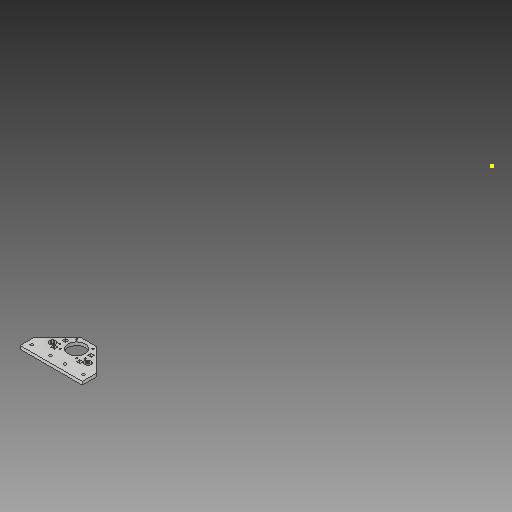
# Autodesk Inventor part: Rear Z Motor Mount
Saved by Autodesk Inventor 2018 (Build 220112000, 112)
## iProperties
Created: 2016-07-25
Part Number: Rear Z Motor Mount
Material: Generic
Document SubType Name: Modeling
Designer: User
Density: 1 g/cm^3
Appearance: Default
Author: User
Autodesk Inventor part; units mm, degrees
ref_plane "YZ Plane" through (0, 0, 0) normal (1, 0, 0) x (0, 1, 0)
ref_plane "XZ Plane" through (0, 0, 0) normal (0, 1, 0) x (-1, 0, 0)
ref_plane "XY Plane" through (0, 0, 0) normal (0, 0, 1) x (1, 0, 0)
sketch "Sketch1" plane through (0, 0, 0) normal (0, 1, 0) x (-1, 0, 0)
  line L0 (139.395291, 734.084292) -> (139.145335, 734.709338)
  line L1 (139.145335, 734.709338) -> (138.74531, 735.209285)
  line L2 (138.74531, 735.209285) -> (138.22032, 735.609261)
  line L3 (138.22032, 735.609261) -> (137.620314, 735.859289)
  line L4 (137.620314, 735.859289) -> (136.970314, 735.959304)
  line L5 (136.970314, 735.959304) -> (136.320293, 735.859285)
  line L6 (136.320293, 735.859285) -> (135.720329, 735.609258)
  line L7 (135.720329, 735.609258) -> (135.19531, 735.209292)
  line L8 (135.19531, 735.209292) -> (134.795318, 734.709302)
  line L9 (134.795318, 734.709302) -> (134.545299, 734.084298)
  line L10 (134.545299, 734.084298) -> (134.470282, 733.434297)
  line L11 (134.470282, 733.434297) -> (134.54536, 732.784303)
  line L12 (134.54536, 732.784303) -> (134.795378, 732.184363)
  line L13 (134.795378, 732.184363) -> (135.19537, 731.659309)
  line L14 (135.19537, 731.659309) -> (135.720373, 731.259323)
  line L15 (135.720373, 731.259323) -> (136.320343, 731.009311)
  line L16 (136.320343, 731.009311) -> (136.970367, 730.934291)
  line L17 (136.970367, 730.934291) -> (137.620418, 731.009376)
  line L18 (137.620418, 731.009376) -> (138.220418, 731.259419)
  line L19 (138.220418, 731.259419) -> (138.745325, 731.659299)
  line L20 (138.745325, 731.659299) -> (139.145329, 732.184326)
  line L21 (139.145329, 732.184326) -> (139.395338, 732.784288)
  line L22 (139.395338, 732.784288) -> (139.49533, 733.434137)
  line L23 (139.49533, 733.434137) -> (139.395291, 734.084292)
  line L24 (109.14464, 718.809311) -> (109.145998, 712.609302)
  line L25 (109.145998, 712.609302) -> (115.545973, 712.610704)
  line L26 (115.545973, 712.610704) -> (115.544615, 718.810713)
  line L27 (115.544615, 718.810713) -> (109.14464, 718.809311)
  line L28 (105.170214, 713.534161) -> (105.020247, 713.909169)
  line L29 (105.020247, 713.909169) -> (104.77027, 714.234177)
  line L30 (104.77027, 714.234177) -> (104.445291, 714.484219)
  line L31 (104.445291, 714.484219) -> (104.045334, 714.659273)
  line L32 (104.045334, 714.659273) -> (103.645324, 714.70929)
  line L33 (103.645324, 714.70929) -> (103.245335, 714.65927)
  line L34 (103.245335, 714.65927) -> (102.845343, 714.484247)
  line L35 (102.845343, 714.484247) -> (102.520335, 714.23427)
  line L36 (102.520335, 714.23427) -> (102.270303, 713.909305)
  line L37 (102.270303, 713.909305) -> (102.120296, 713.534313)
  line L38 (102.120296, 713.534313) -> (102.070277, 713.109272)
  line L39 (102.070277, 713.109272) -> (102.120296, 712.709294)
  line L40 (102.120296, 712.709294) -> (102.270268, 712.309311)
  line L41 (102.270268, 712.309311) -> (102.520266, 711.984276)
  line L42 (102.520266, 711.984276) -> (102.84521, 711.73426)
  line L43 (102.84521, 711.73426) -> (103.245165, 711.584114)
  line L44 (103.245165, 711.584114) -> (103.645165, 711.534098)
  line L45 (103.645165, 711.534098) -> (104.045186, 711.584122)
  line L46 (104.045186, 711.584122) -> (104.445183, 711.734099)
  line L47 (104.445183, 711.734099) -> (104.770183, 711.984071)
  line L48 (104.770183, 711.984071) -> (105.020236, 712.309063)
  line L49 (105.020236, 712.309063) -> (105.17037, 712.708985)
  line L50 (105.17037, 712.708985) -> (105.245245, 713.108394)
  line L51 (105.245245, 713.108394) -> (105.170214, 713.534161)
  line L52 (103.59529, 701.759382) -> (101.995303, 705.60938)
  line L53 (101.995303, 705.60938) -> (99.470328, 708.934371)
  line L54 (99.470328, 708.934371) -> (96.145337, 711.484388)
  line L55 (96.145337, 711.484388) -> (92.295319, 713.05936)
  line L56 (92.295319, 713.05936) -> (88.145309, 713.609327)
  line L57 (88.145309, 713.609327) -> (83.995304, 713.059318)
  line L58 (83.995304, 713.059318) -> (80.14528, 711.484306)
  line L59 (80.14528, 711.484306) -> (76.820289, 708.93429)
  line L60 (76.820289, 708.93429) -> (74.295314, 705.609299)
  line L61 (74.295314, 705.609299) -> (72.695283, 701.759319)
  line L62 (72.695283, 701.759319) -> (72.145316, 697.609313)
  line L63 (72.145316, 697.609313) -> (72.695283, 693.484285)
  line L64 (72.695283, 693.484285) -> (74.295314, 689.609285)
  line L65 (74.295314, 689.609285) -> (76.820289, 686.309314)
  line L66 (76.820289, 686.309314) -> (80.14528, 683.759298)
  line L67 (80.14528, 683.759298) -> (83.995282, 682.159257)
  line L68 (83.995282, 682.159257) -> (88.145293, 681.60929)
  line L69 (88.145293, 681.60929) -> (92.295298, 682.159299)
  line L70 (92.295298, 682.159299) -> (96.1453, 683.759288)
  line L71 (96.1453, 683.759288) -> (99.470291, 686.309304)
  line L72 (99.470291, 686.309304) -> (101.995266, 689.609275)
  line L73 (101.995266, 689.609275) -> (103.595297, 693.484276)
  line L74 (103.595297, 693.484276) -> (104.14532, 697.609224)
  line L75 (104.14532, 697.609224) -> (103.59529, 701.759382)
  line L76 (113.895233, 705.508847) -> (113.745267, 705.883856)
  line L77 (113.745267, 705.883856) -> (113.520146, 706.209334)
  line L78 (113.520146, 706.209334) -> (113.195174, 706.459372)
  line L79 (113.195174, 706.459372) -> (112.845114, 706.634306)
  line L80 (112.845114, 706.634306) -> (112.445132, 706.709288)
  line L81 (112.445132, 706.709288) -> (112.045113, 706.684282)
  line L82 (112.045113, 706.684282) -> (111.670099, 706.559312)
  line L83 (111.670099, 706.559312) -> (111.320076, 706.359366)
  line L84 (111.320076, 706.359366) -> (111.045103, 706.059375)
  line L85 (111.045103, 706.059375) -> (110.870168, 705.709315)
  line L86 (110.870168, 705.709315) -> (110.770262, 705.309317)
  line L87 (110.770262, 705.309317) -> (110.77035, 704.909299)
  line L88 (110.77035, 704.909299) -> (110.870426, 704.534322)
  line L89 (110.870426, 704.534322) -> (111.04538, 704.184315)
  line L90 (111.04538, 704.184315) -> (111.320343, 703.884272)
  line L91 (111.320343, 703.884272) -> (111.670328, 703.659241)
  line L92 (111.670328, 703.659241) -> (112.045299, 703.534186)
  line L93 (112.045299, 703.534186) -> (112.445314, 703.50911)
  line L94 (112.445314, 703.50911) -> (112.845294, 703.584062)
  line L95 (112.845294, 703.584062) -> (113.195352, 703.759042)
  line L96 (113.195352, 703.759042) -> (113.520346, 704.009009)
  line L97 (113.520346, 704.009009) -> (113.745232, 704.333827)
  line L98 (113.745232, 704.333827) -> (113.895239, 704.708819)
  line L99 (113.895239, 704.708819) -> (113.945257, 705.108829)
  line L100 (113.945257, 705.108829) -> (113.895233, 705.508847)
  line L101 (109.14464, 697.609313) -> (109.145998, 691.409304)
  line L102 (109.145998, 691.409304) -> (115.545973, 691.410706)
  line L103 (115.545973, 691.410706) -> (115.544615, 697.610715)
  line L104 (115.544615, 697.610715) -> (109.14464, 697.609313)
  line L105 (105.16778, 682.533999) -> (105.017813, 682.909007)
  line L106 (105.017813, 682.909007) -> (104.767857, 683.233987)
  line L107 (104.767857, 683.233987) -> (104.442857, 683.484046)
  line L108 (104.442857, 683.484046) -> (104.0429, 683.6591)
  line L109 (104.0429, 683.6591) -> (103.642836, 683.709124)
  line L110 (103.642836, 683.709124) -> (103.242842, 683.659103)
  line L111 (103.242842, 683.659103) -> (102.84285, 683.48408)
  line L112 (102.84285, 683.48408) -> (102.517822, 683.234087)
  line L113 (102.517822, 683.234087) -> (102.26781, 682.909149)
  line L114 (102.26781, 682.909149) -> (102.117803, 682.534157)
  line L115 (102.117803, 682.534157) -> (102.042746, 682.108654)
  line L116 (102.042746, 682.108654) -> (102.117675, 681.708798)
  line L117 (102.117675, 681.708798) -> (102.267647, 681.308815)
  line L118 (102.267647, 681.308815) -> (102.517645, 680.983781)
  line L119 (102.517645, 680.983781) -> (102.84261, 680.733749)
  line L120 (102.84261, 680.733749) -> (103.242551, 680.583608)
  line L121 (103.242551, 680.583608) -> (103.642546, 680.533593)
  line L122 (103.642546, 680.533593) -> (104.042561, 680.583616)
  line L123 (104.042561, 680.583616) -> (104.442544, 680.733588)
  line L124 (104.442544, 680.733588) -> (104.767565, 680.983576)
  line L125 (104.767565, 680.983576) -> (105.017618, 681.308568)
  line L126 (105.017618, 681.308568) -> (105.167752, 681.70849)
  line L127 (105.167752, 681.70849) -> (105.242752, 682.108567)
  line L128 (105.242752, 682.108567) -> (105.16778, 682.533999)
  line L129 (74.171005, 682.534425) -> (74.021036, 682.90944)
  line L130 (74.021036, 682.90944) -> (73.771079, 683.234421)
  line L131 (73.771079, 683.234421) -> (73.446094, 683.484469)
  line L132 (73.446094, 683.484469) -> (73.0461, 683.659538)
  line L133 (73.0461, 683.659538) -> (72.646127, 683.709551)
  line L134 (72.646127, 683.709551) -> (72.246112, 683.659528)
  line L135 (72.246112, 683.659528) -> (71.846138, 683.484513)
  line L136 (71.846138, 683.484513) -> (71.521096, 683.234509)
  line L137 (71.521096, 683.234509) -> (71.271076, 682.909561)
  line L138 (71.271076, 682.909561) -> (71.121072, 682.534576)
  line L139 (71.121072, 682.534576) -> (71.046082, 682.109455)
  line L140 (71.046082, 682.109455) -> (71.121043, 681.70943)
  line L141 (71.121043, 681.70943) -> (71.271013, 681.309455)
  line L142 (71.271013, 681.309455) -> (71.521019, 680.98441)
  line L143 (71.521019, 680.98441) -> (71.845997, 680.734367)
  line L144 (71.845997, 680.734367) -> (72.245919, 680.584234)
  line L145 (72.245919, 680.584234) -> (72.645863, 680.534224)
  line L146 (72.645863, 680.534224) -> (73.045836, 680.584243)
  line L147 (73.045836, 680.584243) -> (73.445857, 680.734229)
  line L148 (73.445857, 680.734229) -> (73.770864, 680.984206)
  line L149 (73.770864, 680.984206) -> (74.020917, 681.309198)
  line L150 (74.020917, 681.309198) -> (74.171053, 681.709127)
  line L151 (74.171053, 681.709127) -> (74.245995, 682.108893)
  line L152 (74.245995, 682.108893) -> (74.171005, 682.534425)
  line L153 (60.744623, 697.609313) -> (60.745981, 691.409304)
  line L154 (60.745981, 691.409304) -> (67.145601, 691.410706)
  line L155 (67.145601, 691.410706) -> (67.144243, 697.610715)
  line L156 (67.144243, 697.610715) -> (60.744623, 697.609313)
  line L157 (65.445222, 705.708927) -> (65.245261, 706.058976)
  line L158 (65.245261, 706.058976) -> (64.970319, 706.358996)
  line L159 (64.970319, 706.358996) -> (64.620368, 706.559031)
  line L160 (64.620368, 706.559031) -> (64.245365, 706.684097)
  line L161 (64.245365, 706.684097) -> (63.845371, 706.709172)
  line L162 (63.845371, 706.709172) -> (63.445342, 706.63421)
  line L163 (63.445342, 706.63421) -> (63.095318, 706.459248)
  line L164 (63.095318, 706.459248) -> (62.770303, 706.209264)
  line L165 (62.770303, 706.209264) -> (62.545319, 705.884305)
  line L166 (62.545319, 705.884305) -> (62.395309, 705.509305)
  line L167 (62.395309, 705.509305) -> (62.34529, 705.109286)
  line L168 (62.34529, 705.109286) -> (62.395309, 704.709311)
  line L169 (62.395309, 704.709311) -> (62.545278, 704.334295)
  line L170 (62.545278, 704.334295) -> (62.770227, 704.009267)
  line L171 (62.770227, 704.009267) -> (63.095178, 703.759245)
  line L172 (63.095178, 703.759245) -> (63.445158, 703.584151)
  line L173 (63.445158, 703.584151) -> (63.845174, 703.509162)
  line L174 (63.845174, 703.509162) -> (64.245172, 703.534167)
  line L175 (64.245172, 703.534167) -> (64.620197, 703.659124)
  line L176 (64.620197, 703.659124) -> (64.970184, 703.884119)
  line L177 (64.970184, 703.884119) -> (65.245179, 704.184133)
  line L178 (65.245179, 704.184133) -> (65.44522, 704.534094)
  line L179 (65.44522, 704.534094) -> (65.545248, 704.909083)
  line L180 (65.545248, 704.909083) -> (65.54516, 705.308937)
  line L181 (65.54516, 705.308937) -> (65.445222, 705.708927)
  line L182 (60.720321, 711.359386) -> (60.120286, 712.809328)
  line L183 (60.120286, 712.809328) -> (59.170321, 714.034334)
  line L184 (59.170321, 714.034334) -> (57.920292, 714.984294)
  line L185 (57.920292, 714.984294) -> (56.470304, 715.584314)
  line L186 (56.470304, 715.584314) -> (54.920313, 715.809279)
  line L187 (54.920313, 715.809279) -> (53.3703, 715.584314)
  line L188 (53.3703, 715.584314) -> (51.920324, 714.984265)
  line L189 (51.920324, 714.984265) -> (50.695291, 714.03428)
  line L190 (50.695291, 714.03428) -> (49.720286, 712.80929)
  line L191 (49.720286, 712.80929) -> (49.120279, 711.359335)
  line L192 (49.120279, 711.359335) -> (48.920291, 709.809301)
  line L193 (48.920291, 709.809301) -> (49.120279, 708.234289)
  line L194 (49.120279, 708.234289) -> (49.720286, 706.809312)
  line L195 (49.720286, 706.809312) -> (50.695291, 705.559302)
  line L196 (50.695291, 705.559302) -> (51.920324, 704.609274)
  line L197 (51.920324, 704.609274) -> (53.370281, 704.009266)
  line L198 (53.370281, 704.009266) -> (54.920295, 703.809281)
  line L199 (54.920295, 703.809281) -> (56.470286, 704.009271)
  line L200 (56.470286, 704.009271) -> (57.920231, 704.609308)
  line L201 (57.920231, 704.609308) -> (59.170193, 705.5594)
  line L202 (59.170193, 705.5594) -> (60.120153, 706.809429)
  line L203 (60.120153, 706.809429) -> (60.720131, 708.234419)
  line L204 (60.720131, 708.234419) -> (60.920304, 709.809457)
  line L205 (60.920304, 709.809457) -> (60.720321, 711.359386)
  line L206 (60.744623, 718.809311) -> (60.745981, 712.609302)
  line L207 (60.745981, 712.609302) -> (67.145956, 712.610704)
  line L208 (67.145956, 712.610704) -> (67.144598, 718.810713)
  line L209 (67.144598, 718.810713) -> (60.744623, 718.809311)
  line L210 (74.170237, 713.534159) -> (74.020268, 713.909175)
  line L211 (74.020268, 713.909175) -> (73.77029, 714.234182)
  line L212 (73.77029, 714.234182) -> (73.445325, 714.484214)
  line L213 (73.445325, 714.484214) -> (73.045332, 714.659284)
  line L214 (73.045332, 714.659284) -> (72.645364, 714.709296)
  line L215 (72.645364, 714.709296) -> (72.245354, 714.659273)
  line L216 (72.245354, 714.659273) -> (71.84538, 714.484258)
  line L217 (71.84538, 714.484258) -> (71.520359, 714.23427)
  line L218 (71.520359, 714.23427) -> (71.270319, 713.909295)
  line L219 (71.270319, 713.909295) -> (71.120314, 713.53431)
  line L220 (71.120314, 713.53431) -> (71.070296, 713.109272)
  line L221 (71.070296, 713.109272) -> (71.120314, 712.709296)
  line L222 (71.120314, 712.709296) -> (71.270284, 712.309321)
  line L223 (71.270284, 712.309321) -> (71.52029, 711.984276)
  line L224 (71.52029, 711.984276) -> (71.845248, 711.734249)
  line L225 (71.845248, 711.734249) -> (72.245184, 711.58411)
  line L226 (72.245184, 711.58411) -> (72.645205, 711.534091)
  line L227 (72.645205, 711.534091) -> (73.045183, 711.58411)
  line L228 (73.045183, 711.58411) -> (73.445218, 711.734102)
  line L229 (73.445218, 711.734102) -> (73.770204, 711.984063)
  line L230 (73.770204, 711.984063) -> (74.020258, 712.309055)
  line L231 (74.020258, 712.309055) -> (74.170394, 712.708984)
  line L232 (74.170394, 712.708984) -> (74.245268, 713.108391)
  line L233 (74.245268, 713.108391) -> (74.170237, 713.534159)
  line L234 (76.595279, 734.084304) -> (76.345325, 734.709343)
  line L235 (76.345325, 734.709343) -> (75.9453, 735.20929)
  line L236 (75.9453, 735.20929) -> (75.420297, 735.609276)
  line L237 (75.420297, 735.609276) -> (74.820291, 735.859304)
  line L238 (74.820291, 735.859304) -> (74.170311, 735.959315)
  line L239 (74.170311, 735.959315) -> (73.520311, 735.8593)
  line L240 (73.520311, 735.8593) -> (72.920297, 735.609251)
  line L241 (72.920297, 735.609251) -> (72.395278, 735.209286)
  line L242 (72.395278, 735.209286) -> (71.995303, 734.709317)
  line L243 (71.995303, 734.709317) -> (71.745278, 734.084298)
  line L244 (71.745278, 734.084298) -> (71.670261, 733.434297)
  line L245 (71.670261, 733.434297) -> (71.745339, 732.784303)
  line L246 (71.745339, 732.784303) -> (71.995364, 732.184347)
  line L247 (71.995364, 732.184347) -> (72.395339, 731.659315)
  line L248 (72.395339, 731.659315) -> (72.920342, 731.259329)
  line L249 (72.920342, 731.259329) -> (73.520349, 731.009301)
  line L250 (73.520349, 731.009301) -> (74.170352, 730.934284)
  line L251 (74.170352, 730.934284) -> (74.820324, 731.009359)
  line L252 (74.820324, 731.009359) -> (75.420324, 731.259402)
  line L253 (75.420324, 731.259402) -> (75.945286, 731.659324)
  line L254 (75.945286, 731.659324) -> (76.34529, 732.184351)
  line L255 (76.34529, 732.184351) -> (76.595297, 732.784306)
  line L256 (76.595297, 732.784306) -> (76.695302, 733.434247)
  line L257 (76.695302, 733.434247) -> (76.595279, 734.084304)
  line L258 (104.570192, 734.084233) -> (104.320241, 734.709264)
  line L259 (104.320241, 734.709264) -> (103.920208, 735.209222)
  line L260 (103.920208, 735.209222) -> (103.395205, 735.609208)
  line L261 (103.395205, 735.609208) -> (102.770266, 735.859201)
  line L262 (102.770266, 735.859201) -> (102.120287, 735.959212)
  line L263 (102.120287, 735.959212) -> (101.470244, 735.859191)
  line L264 (101.470244, 735.859191) -> (100.845246, 735.609253)
  line L265 (100.845246, 735.609253) -> (100.320228, 735.209288)
  line L266 (100.320228, 735.209288) -> (99.920235, 734.709298)
  line L267 (99.920235, 734.709298) -> (99.670213, 734.084286)
  line L268 (99.670213, 734.084286) -> (99.570198, 733.434286)
  line L269 (99.570198, 733.434286) -> (99.670213, 732.784286)
  line L270 (99.670213, 732.784286) -> (99.920235, 732.184338)
  line L271 (99.920235, 732.184338) -> (100.320226, 731.659284)
  line L272 (100.320226, 731.659284) -> (100.845229, 731.259298)
  line L273 (100.845229, 731.259298) -> (101.4702, 731.009293)
  line L274 (101.4702, 731.009293) -> (102.120246, 730.934271)
  line L275 (102.120246, 730.934271) -> (102.770221, 731.009347)
  line L276 (102.770221, 731.009347) -> (103.395237, 731.259292)
  line L277 (103.395237, 731.259292) -> (103.920134, 731.659163)
  line L278 (103.920134, 731.659163) -> (104.320146, 732.184201)
  line L279 (104.320146, 732.184201) -> (104.570149, 732.784148)
  line L280 (104.570149, 732.784148) -> (104.670192, 733.434331)
  line L281 (104.670192, 733.434331) -> (104.570192, 734.084233)
  line L282 (41.745244, 734.084338) -> (41.495293, 734.70937)
  line L283 (41.495293, 734.70937) -> (41.095291, 735.209288)
  line L284 (41.095291, 735.209288) -> (40.570288, 735.609274)
  line L285 (40.570288, 735.609274) -> (39.970281, 735.859302)
  line L286 (39.970281, 735.859302) -> (39.320302, 735.959314)
  line L287 (39.320302, 735.959314) -> (38.670302, 735.859299)
  line L288 (38.670302, 735.859299) -> (38.070302, 735.609256)
  line L289 (38.070302, 735.609256) -> (37.545297, 735.209301)
  line L290 (37.545297, 735.209301) -> (37.145321, 734.709331)
  line L291 (37.145321, 734.709331) -> (36.895293, 734.084305)
  line L292 (36.895293, 734.084305) -> (36.795278, 733.434302)
  line L293 (36.795278, 733.434302) -> (36.895293, 732.784298)
  line L294 (36.895293, 732.784298) -> (37.145321, 732.184335)
  line L295 (37.145321, 732.184335) -> (37.545297, 731.659302)
  line L296 (37.545297, 731.659302) -> (38.070286, 731.259327)
  line L297 (38.070286, 731.259327) -> (38.670292, 731.009299)
  line L298 (38.670292, 731.009299) -> (39.320296, 730.934282)
  line L299 (39.320296, 730.934282) -> (39.970271, 731.009358)
  line L300 (39.970271, 731.009358) -> (40.570271, 731.259401)
  line L301 (40.570271, 731.259401) -> (41.09529, 731.659366)
  line L302 (41.09529, 731.659366) -> (41.495302, 732.184403)
  line L303 (41.495302, 732.184403) -> (41.745305, 732.78435)
  line L304 (41.745305, 732.78435) -> (41.820321, 733.434347)
  line L305 (41.820321, 733.434347) -> (41.745244, 734.084338)
  line L306 (29.317325, 745.634246) -> (29.323282, 718.434313)
  line L307 (29.323282, 718.434313) -> (72.657773, 675.118798)
  line L308 (72.657773, 675.118798) -> (103.657753, 675.125587)
  line L309 (103.657753, 675.125587) -> (146.973268, 718.460078)
  line L310 (146.973268, 718.460078) -> (146.967311, 745.66001)
  line L311 (146.967311, 745.66001) -> (29.317325, 745.634246)
  line L312 (127.170308, 711.359328) -> (126.570264, 712.809292)
  line L313 (126.570264, 712.809292) -> (125.595227, 714.03429)
  line L314 (125.595227, 714.03429) -> (124.370208, 714.984308)
  line L315 (124.370208, 714.984308) -> (122.920216, 715.584329)
  line L316 (122.920216, 715.584329) -> (121.370225, 715.809294)
  line L317 (121.370225, 715.809294) -> (119.820212, 715.584329)
  line L318 (119.820212, 715.584329) -> (118.370251, 714.984286)
  line L319 (118.370251, 714.984286) -> (117.120289, 714.034195)
  line L320 (117.120289, 714.034195) -> (116.170282, 712.809189)
  line L321 (116.170282, 712.809189) -> (115.570267, 711.359212)
  line L322 (115.570267, 711.359212) -> (115.370283, 709.809215)
  line L323 (115.370283, 709.809215) -> (115.570272, 708.234198)
  line L324 (115.570272, 708.234198) -> (116.170287, 706.809199)
  line L325 (116.170287, 706.809199) -> (117.120379, 705.559237)
  line L326 (117.120379, 705.559237) -> (118.370408, 704.609277)
  line L327 (118.370408, 704.609277) -> (119.820381, 704.009263)
  line L328 (119.820381, 704.009263) -> (121.370394, 703.809278)
  line L329 (121.370394, 703.809278) -> (122.920385, 704.009269)
  line L330 (122.920385, 704.009269) -> (124.370365, 704.60932)
  line L331 (124.370365, 704.60932) -> (125.595384, 705.559294)
  line L332 (125.595384, 705.559294) -> (126.570146, 706.809314)
  line L333 (126.570146, 706.809314) -> (127.170133, 708.234325)
  line L334 (127.170133, 708.234325) -> (127.370301, 709.809322)
  line L335 (127.370301, 709.809322) -> (127.170308, 711.359328)
  point P0 (0, 0)
  constraints: 672 end point, 122 parallel, 97 perpendicular
extrude "Extrusion1" add sketch "Sketch1" along normal blind 6 contours L281 L280 L279 L278 L277 L276 L275 L274 L273 L272 L271 L270 L269 L268 L267 L266 L265 L264 L263 L262 L261 L260 L259 L258 | L311 L310 L309 L308 L307 L306
sketch "Sketch2" plane through (0, 0, 0) normal (0, -1, 0) x (1, 0, 0)
  line L0 (-104.14532, 697.609224) -> (-103.59529, 701.759382)
  line L1 (-103.59529, 701.759382) -> (-101.995303, 705.60938)
  line L2 (-101.995303, 705.60938) -> (-99.470328, 708.934371)
  line L3 (-99.470328, 708.934371) -> (-96.145337, 711.484388)
  line L4 (-96.145337, 711.484388) -> (-92.295319, 713.05936)
  line L5 (-92.295319, 713.05936) -> (-88.145309, 713.609327)
  line L6 (-88.145309, 713.609327) -> (-83.995304, 713.059318)
  line L7 (-83.995304, 713.059318) -> (-80.14528, 711.484306)
  line L8 (-80.14528, 711.484306) -> (-76.820289, 708.93429)
  line L9 (-76.820289, 708.93429) -> (-74.295314, 705.609299)
  line L10 (-74.295314, 705.609299) -> (-72.695283, 701.759319)
  line L11 (-72.695283, 701.759319) -> (-72.145316, 697.609313)
  line L12 (-72.145316, 697.609313) -> (-72.695283, 693.484285)
  line L13 (-72.695283, 693.484285) -> (-74.295314, 689.609285)
  line L14 (-74.295314, 689.609285) -> (-76.820289, 686.309314)
  line L15 (-76.820289, 686.309314) -> (-80.14528, 683.759298)
  line L16 (-80.14528, 683.759298) -> (-83.995282, 682.159257)
  line L17 (-83.995282, 682.159257) -> (-88.145293, 681.60929)
  line L18 (-88.145293, 681.60929) -> (-92.295298, 682.159299)
  line L19 (-92.295298, 682.159299) -> (-96.1453, 683.759288)
  line L20 (-96.1453, 683.759288) -> (-99.470291, 686.309304)
  line L21 (-99.470291, 686.309304) -> (-101.995266, 689.609275)
  line L22 (-101.995266, 689.609275) -> (-103.595297, 693.484276)
  line L23 (-103.595297, 693.484276) -> (-104.14532, 697.609224)
  line L24 (-127.370301, 709.809322) -> (-127.170308, 711.359328)
  line L25 (-127.170308, 711.359328) -> (-126.570264, 712.809292)
  line L26 (-126.570264, 712.809292) -> (-125.595227, 714.03429)
  line L27 (-125.595227, 714.03429) -> (-124.370208, 714.984308)
  line L28 (-124.370208, 714.984308) -> (-122.920216, 715.584329)
  line L29 (-122.920216, 715.584329) -> (-121.370225, 715.809294)
  line L30 (-121.370225, 715.809294) -> (-119.820212, 715.584329)
  line L31 (-119.820212, 715.584329) -> (-118.370251, 714.984286)
  line L32 (-118.370251, 714.984286) -> (-117.120289, 714.034195)
  line L33 (-117.120289, 714.034195) -> (-116.170282, 712.809189)
  line L34 (-116.170282, 712.809189) -> (-115.570267, 711.359212)
  line L35 (-115.570267, 711.359212) -> (-115.370283, 709.809215)
  line L36 (-115.370283, 709.809215) -> (-115.570272, 708.234198)
  line L37 (-115.570272, 708.234198) -> (-116.170287, 706.809199)
  line L38 (-116.170287, 706.809199) -> (-117.120379, 705.559237)
  line L39 (-117.120379, 705.559237) -> (-118.370408, 704.609277)
  line L40 (-118.370408, 704.609277) -> (-119.820381, 704.009263)
  line L41 (-119.820381, 704.009263) -> (-121.370394, 703.809278)
  line L42 (-121.370394, 703.809278) -> (-122.920385, 704.009269)
  line L43 (-122.920385, 704.009269) -> (-124.370365, 704.60932)
  line L44 (-124.370365, 704.60932) -> (-125.595384, 705.559294)
  line L45 (-125.595384, 705.559294) -> (-126.570146, 706.809314)
  line L46 (-126.570146, 706.809314) -> (-127.170133, 708.234325)
  line L47 (-127.170133, 708.234325) -> (-127.370301, 709.809322)
  line L48 (-60.920304, 709.809457) -> (-60.720321, 711.359386)
  line L49 (-60.720321, 711.359386) -> (-60.120286, 712.809328)
  line L50 (-60.120286, 712.809328) -> (-59.170321, 714.034334)
  line L51 (-59.170321, 714.034334) -> (-57.920292, 714.984294)
  line L52 (-57.920292, 714.984294) -> (-56.470304, 715.584314)
  line L53 (-56.470304, 715.584314) -> (-54.920313, 715.809279)
  line L54 (-54.920313, 715.809279) -> (-53.3703, 715.584314)
  line L55 (-53.3703, 715.584314) -> (-51.920324, 714.984265)
  line L56 (-51.920324, 714.984265) -> (-50.695291, 714.03428)
  line L57 (-50.695291, 714.03428) -> (-49.720286, 712.80929)
  line L58 (-49.720286, 712.80929) -> (-49.120279, 711.359335)
  line L59 (-49.120279, 711.359335) -> (-48.920291, 709.809301)
  line L60 (-48.920291, 709.809301) -> (-49.120279, 708.234289)
  line L61 (-49.120279, 708.234289) -> (-49.720286, 706.809312)
  line L62 (-49.720286, 706.809312) -> (-50.695291, 705.559302)
  line L63 (-50.695291, 705.559302) -> (-51.920324, 704.609274)
  line L64 (-51.920324, 704.609274) -> (-53.370281, 704.009266)
  line L65 (-53.370281, 704.009266) -> (-54.920295, 703.809281)
  line L66 (-54.920295, 703.809281) -> (-56.470286, 704.009271)
  line L67 (-56.470286, 704.009271) -> (-57.920231, 704.609308)
  line L68 (-57.920231, 704.609308) -> (-59.170193, 705.5594)
  line L69 (-59.170193, 705.5594) -> (-60.120153, 706.809429)
  line L70 (-60.120153, 706.809429) -> (-60.720131, 708.234419)
  line L71 (-60.720131, 708.234419) -> (-60.920304, 709.809457)
  line L72 (-67.144598, 718.810713) -> (-60.744623, 718.809311)
  line L73 (-60.744623, 718.809311) -> (-60.745981, 712.609302)
  line L74 (-60.745981, 712.609302) -> (-67.145956, 712.610704)
  line L75 (-67.145956, 712.610704) -> (-67.144598, 718.810713)
  line L76 (-115.544615, 697.610715) -> (-109.14464, 697.609313)
  line L77 (-109.14464, 697.609313) -> (-109.145998, 691.409304)
  line L78 (-109.145998, 691.409304) -> (-115.545973, 691.410706)
  line L79 (-115.545973, 691.410706) -> (-115.544615, 697.610715)
  line L80 (-115.544615, 718.810713) -> (-109.14464, 718.809311)
  line L81 (-109.14464, 718.809311) -> (-109.145998, 712.609302)
  line L82 (-109.145998, 712.609302) -> (-115.545973, 712.610704)
  line L83 (-115.545973, 712.610704) -> (-115.544615, 718.810713)
  line L84 (-67.144243, 697.610715) -> (-60.744623, 697.609313)
  line L85 (-60.744623, 697.609313) -> (-60.745981, 691.409304)
  line L86 (-60.745981, 691.409304) -> (-67.145601, 691.410706)
  line L87 (-67.145601, 691.410706) -> (-67.144243, 697.610715)
  line L88 (-139.49533, 733.434137) -> (-139.395291, 734.084292)
  line L89 (-139.395291, 734.084292) -> (-139.145335, 734.709338)
  line L90 (-139.145335, 734.709338) -> (-138.74531, 735.209285)
  line L91 (-138.74531, 735.209285) -> (-138.22032, 735.609261)
  line L92 (-138.22032, 735.609261) -> (-137.620314, 735.859289)
  line L93 (-137.620314, 735.859289) -> (-136.970314, 735.959304)
  line L94 (-136.970314, 735.959304) -> (-136.320293, 735.859285)
  line L95 (-136.320293, 735.859285) -> (-135.720329, 735.609258)
  line L96 (-135.720329, 735.609258) -> (-135.19531, 735.209292)
  line L97 (-135.19531, 735.209292) -> (-134.795318, 734.709302)
  line L98 (-134.795318, 734.709302) -> (-134.545299, 734.084298)
  line L99 (-134.545299, 734.084298) -> (-134.470282, 733.434297)
  line L100 (-134.470282, 733.434297) -> (-134.54536, 732.784303)
  line L101 (-134.54536, 732.784303) -> (-134.795378, 732.184363)
  line L102 (-134.795378, 732.184363) -> (-135.19537, 731.659309)
  line L103 (-135.19537, 731.659309) -> (-135.720373, 731.259323)
  line L104 (-135.720373, 731.259323) -> (-136.320343, 731.009311)
  line L105 (-136.320343, 731.009311) -> (-136.970367, 730.934291)
  line L106 (-136.970367, 730.934291) -> (-137.620418, 731.009376)
  line L107 (-137.620418, 731.009376) -> (-138.220418, 731.259419)
  line L108 (-138.220418, 731.259419) -> (-138.745325, 731.659299)
  line L109 (-138.745325, 731.659299) -> (-139.145329, 732.184326)
  line L110 (-139.145329, 732.184326) -> (-139.395338, 732.784288)
  line L111 (-139.395338, 732.784288) -> (-139.49533, 733.434137)
  line L112 (-41.820321, 733.434347) -> (-41.745244, 734.084338)
  line L113 (-41.745244, 734.084338) -> (-41.495293, 734.70937)
  line L114 (-41.495293, 734.70937) -> (-41.095291, 735.209288)
  line L115 (-41.095291, 735.209288) -> (-40.570288, 735.609274)
  line L116 (-40.570288, 735.609274) -> (-39.970281, 735.859302)
  line L117 (-39.970281, 735.859302) -> (-39.320302, 735.959314)
  line L118 (-39.320302, 735.959314) -> (-38.670302, 735.859299)
  line L119 (-38.670302, 735.859299) -> (-38.070302, 735.609256)
  line L120 (-38.070302, 735.609256) -> (-37.545297, 735.209301)
  line L121 (-37.545297, 735.209301) -> (-37.145321, 734.709331)
  line L122 (-37.145321, 734.709331) -> (-36.895293, 734.084305)
  line L123 (-36.895293, 734.084305) -> (-36.795278, 733.434302)
  line L124 (-36.795278, 733.434302) -> (-36.895293, 732.784298)
  line L125 (-36.895293, 732.784298) -> (-37.145321, 732.184335)
  line L126 (-37.145321, 732.184335) -> (-37.545297, 731.659302)
  line L127 (-37.545297, 731.659302) -> (-38.070286, 731.259327)
  line L128 (-38.070286, 731.259327) -> (-38.670292, 731.009299)
  line L129 (-38.670292, 731.009299) -> (-39.320296, 730.934282)
  line L130 (-39.320296, 730.934282) -> (-39.970271, 731.009358)
  line L131 (-39.970271, 731.009358) -> (-40.570271, 731.259401)
  line L132 (-40.570271, 731.259401) -> (-41.09529, 731.659366)
  line L133 (-41.09529, 731.659366) -> (-41.495302, 732.184403)
  line L134 (-41.495302, 732.184403) -> (-41.745305, 732.78435)
  line L135 (-41.745305, 732.78435) -> (-41.820321, 733.434347)
  line L136 (-76.695302, 733.434247) -> (-76.595279, 734.084304)
  line L137 (-76.595279, 734.084304) -> (-76.345325, 734.709343)
  line L138 (-76.345325, 734.709343) -> (-75.9453, 735.20929)
  line L139 (-75.9453, 735.20929) -> (-75.420297, 735.609276)
  line L140 (-75.420297, 735.609276) -> (-74.820291, 735.859304)
  line L141 (-74.820291, 735.859304) -> (-74.170311, 735.959315)
  line L142 (-74.170311, 735.959315) -> (-73.520311, 735.8593)
  line L143 (-73.520311, 735.8593) -> (-72.920297, 735.609251)
  line L144 (-72.920297, 735.609251) -> (-72.395278, 735.209286)
  line L145 (-72.395278, 735.209286) -> (-71.995303, 734.709317)
  line L146 (-71.995303, 734.709317) -> (-71.745278, 734.084298)
  line L147 (-71.745278, 734.084298) -> (-71.670261, 733.434297)
  line L148 (-71.670261, 733.434297) -> (-71.745339, 732.784303)
  line L149 (-71.745339, 732.784303) -> (-71.995364, 732.184347)
  line L150 (-71.995364, 732.184347) -> (-72.395339, 731.659315)
  line L151 (-72.395339, 731.659315) -> (-72.920342, 731.259329)
  line L152 (-72.920342, 731.259329) -> (-73.520349, 731.009301)
  line L153 (-73.520349, 731.009301) -> (-74.170352, 730.934284)
  line L154 (-74.170352, 730.934284) -> (-74.820324, 731.009359)
  line L155 (-74.820324, 731.009359) -> (-75.420324, 731.259402)
  line L156 (-75.420324, 731.259402) -> (-75.945286, 731.659324)
  line L157 (-75.945286, 731.659324) -> (-76.34529, 732.184351)
  line L158 (-76.34529, 732.184351) -> (-76.595297, 732.784306)
  line L159 (-76.595297, 732.784306) -> (-76.695302, 733.434247)
  line L160 (-65.54516, 705.308937) -> (-65.445222, 705.708927)
  line L161 (-65.445222, 705.708927) -> (-65.245261, 706.058976)
  line L162 (-65.245261, 706.058976) -> (-64.970319, 706.358996)
  line L163 (-64.970319, 706.358996) -> (-64.620368, 706.559031)
  line L164 (-64.620368, 706.559031) -> (-64.245365, 706.684097)
  line L165 (-64.245365, 706.684097) -> (-63.845371, 706.709172)
  line L166 (-63.845371, 706.709172) -> (-63.445342, 706.63421)
  line L167 (-63.445342, 706.63421) -> (-63.095318, 706.459248)
  line L168 (-63.095318, 706.459248) -> (-62.770303, 706.209264)
  line L169 (-62.770303, 706.209264) -> (-62.545319, 705.884305)
  line L170 (-62.545319, 705.884305) -> (-62.395309, 705.509305)
  line L171 (-62.395309, 705.509305) -> (-62.34529, 705.109286)
  line L172 (-62.34529, 705.109286) -> (-62.395309, 704.709311)
  line L173 (-62.395309, 704.709311) -> (-62.545278, 704.334295)
  line L174 (-62.545278, 704.334295) -> (-62.770227, 704.009267)
  line L175 (-62.770227, 704.009267) -> (-63.095178, 703.759245)
  line L176 (-63.095178, 703.759245) -> (-63.445158, 703.584151)
  line L177 (-63.445158, 703.584151) -> (-63.845174, 703.509162)
  line L178 (-63.845174, 703.509162) -> (-64.245172, 703.534167)
  line L179 (-64.245172, 703.534167) -> (-64.620197, 703.659124)
  line L180 (-64.620197, 703.659124) -> (-64.970184, 703.884119)
  line L181 (-64.970184, 703.884119) -> (-65.245179, 704.184133)
  line L182 (-65.245179, 704.184133) -> (-65.44522, 704.534094)
  line L183 (-65.44522, 704.534094) -> (-65.545248, 704.909083)
  line L184 (-65.545248, 704.909083) -> (-65.54516, 705.308937)
  line L185 (-113.945257, 705.108829) -> (-113.895233, 705.508847)
  line L186 (-113.895233, 705.508847) -> (-113.745267, 705.883856)
  line L187 (-113.745267, 705.883856) -> (-113.520146, 706.209334)
  line L188 (-113.520146, 706.209334) -> (-113.195174, 706.459372)
  line L189 (-113.195174, 706.459372) -> (-112.845114, 706.634306)
  line L190 (-112.845114, 706.634306) -> (-112.445132, 706.709288)
  line L191 (-112.445132, 706.709288) -> (-112.045113, 706.684282)
  line L192 (-112.045113, 706.684282) -> (-111.670099, 706.559312)
  line L193 (-111.670099, 706.559312) -> (-111.320076, 706.359366)
  line L194 (-111.320076, 706.359366) -> (-111.045103, 706.059375)
  line L195 (-111.045103, 706.059375) -> (-110.870168, 705.709315)
  line L196 (-110.870168, 705.709315) -> (-110.770262, 705.309317)
  line L197 (-110.770262, 705.309317) -> (-110.77035, 704.909299)
  line L198 (-110.77035, 704.909299) -> (-110.870426, 704.534322)
  line L199 (-110.870426, 704.534322) -> (-111.04538, 704.184315)
  line L200 (-111.04538, 704.184315) -> (-111.320343, 703.884272)
  line L201 (-111.320343, 703.884272) -> (-111.670328, 703.659241)
  line L202 (-111.670328, 703.659241) -> (-112.045299, 703.534186)
  line L203 (-112.045299, 703.534186) -> (-112.445314, 703.50911)
  line L204 (-112.445314, 703.50911) -> (-112.845294, 703.584062)
  line L205 (-112.845294, 703.584062) -> (-113.195352, 703.759042)
  line L206 (-113.195352, 703.759042) -> (-113.520346, 704.009009)
  line L207 (-113.520346, 704.009009) -> (-113.745232, 704.333827)
  line L208 (-113.745232, 704.333827) -> (-113.895239, 704.708819)
  line L209 (-113.895239, 704.708819) -> (-113.945257, 705.108829)
  line L210 (-105.242752, 682.108567) -> (-105.16778, 682.533999)
  line L211 (-105.16778, 682.533999) -> (-105.017813, 682.909007)
  line L212 (-105.017813, 682.909007) -> (-104.767857, 683.233987)
  line L213 (-104.767857, 683.233987) -> (-104.442857, 683.484046)
  line L214 (-104.442857, 683.484046) -> (-104.0429, 683.6591)
  line L215 (-104.0429, 683.6591) -> (-103.642836, 683.709124)
  line L216 (-103.642836, 683.709124) -> (-103.242842, 683.659103)
  line L217 (-103.242842, 683.659103) -> (-102.84285, 683.48408)
  line L218 (-102.84285, 683.48408) -> (-102.517822, 683.234087)
  line L219 (-102.517822, 683.234087) -> (-102.26781, 682.909149)
  line L220 (-102.26781, 682.909149) -> (-102.117803, 682.534157)
  line L221 (-102.117803, 682.534157) -> (-102.042746, 682.108654)
  line L222 (-102.042746, 682.108654) -> (-102.117675, 681.708798)
  line L223 (-102.117675, 681.708798) -> (-102.267647, 681.308815)
  line L224 (-102.267647, 681.308815) -> (-102.517645, 680.983781)
  line L225 (-102.517645, 680.983781) -> (-102.84261, 680.733749)
  line L226 (-102.84261, 680.733749) -> (-103.242551, 680.583608)
  line L227 (-103.242551, 680.583608) -> (-103.642546, 680.533593)
  line L228 (-103.642546, 680.533593) -> (-104.042561, 680.583616)
  line L229 (-104.042561, 680.583616) -> (-104.442544, 680.733588)
  line L230 (-104.442544, 680.733588) -> (-104.767565, 680.983576)
  line L231 (-104.767565, 680.983576) -> (-105.017618, 681.308568)
  line L232 (-105.017618, 681.308568) -> (-105.167752, 681.70849)
  line L233 (-105.167752, 681.70849) -> (-105.242752, 682.108567)
  line L234 (-74.245995, 682.108893) -> (-74.171005, 682.534425)
  line L235 (-74.171005, 682.534425) -> (-74.021036, 682.90944)
  line L236 (-74.021036, 682.90944) -> (-73.771079, 683.234421)
  line L237 (-73.771079, 683.234421) -> (-73.446094, 683.484469)
  line L238 (-73.446094, 683.484469) -> (-73.0461, 683.659538)
  line L239 (-73.0461, 683.659538) -> (-72.646127, 683.709551)
  line L240 (-72.646127, 683.709551) -> (-72.246112, 683.659528)
  line L241 (-72.246112, 683.659528) -> (-71.846138, 683.484513)
  line L242 (-71.846138, 683.484513) -> (-71.521096, 683.234509)
  line L243 (-71.521096, 683.234509) -> (-71.271076, 682.909561)
  line L244 (-71.271076, 682.909561) -> (-71.121072, 682.534576)
  line L245 (-71.121072, 682.534576) -> (-71.046082, 682.109455)
  line L246 (-71.046082, 682.109455) -> (-71.121043, 681.70943)
  line L247 (-71.121043, 681.70943) -> (-71.271013, 681.309455)
  line L248 (-71.271013, 681.309455) -> (-71.521019, 680.98441)
  line L249 (-71.521019, 680.98441) -> (-71.845997, 680.734367)
  line L250 (-71.845997, 680.734367) -> (-72.245919, 680.584234)
  line L251 (-72.245919, 680.584234) -> (-72.645863, 680.534224)
  line L252 (-72.645863, 680.534224) -> (-73.045836, 680.584243)
  line L253 (-73.045836, 680.584243) -> (-73.445857, 680.734229)
  line L254 (-73.445857, 680.734229) -> (-73.770864, 680.984206)
  line L255 (-73.770864, 680.984206) -> (-74.020917, 681.309198)
  line L256 (-74.020917, 681.309198) -> (-74.171053, 681.709127)
  line L257 (-74.171053, 681.709127) -> (-74.245995, 682.108893)
  line L258 (-74.245268, 713.108391) -> (-74.170237, 713.534159)
  line L259 (-74.170237, 713.534159) -> (-74.020268, 713.909175)
  line L260 (-74.020268, 713.909175) -> (-73.77029, 714.234182)
  line L261 (-73.77029, 714.234182) -> (-73.445325, 714.484214)
  line L262 (-73.445325, 714.484214) -> (-73.045332, 714.659284)
  line L263 (-73.045332, 714.659284) -> (-72.645364, 714.709296)
  line L264 (-72.645364, 714.709296) -> (-72.245354, 714.659273)
  line L265 (-72.245354, 714.659273) -> (-71.84538, 714.484258)
  line L266 (-71.84538, 714.484258) -> (-71.520359, 714.23427)
  line L267 (-71.520359, 714.23427) -> (-71.270319, 713.909295)
  line L268 (-71.270319, 713.909295) -> (-71.120314, 713.53431)
  line L269 (-71.120314, 713.53431) -> (-71.070296, 713.109272)
  line L270 (-71.070296, 713.109272) -> (-71.120314, 712.709296)
  line L271 (-71.120314, 712.709296) -> (-71.270284, 712.309321)
  line L272 (-71.270284, 712.309321) -> (-71.52029, 711.984276)
  line L273 (-71.52029, 711.984276) -> (-71.845248, 711.734249)
  line L274 (-71.845248, 711.734249) -> (-72.245184, 711.58411)
  line L275 (-72.245184, 711.58411) -> (-72.645205, 711.534091)
  line L276 (-72.645205, 711.534091) -> (-73.045183, 711.58411)
  line L277 (-73.045183, 711.58411) -> (-73.445218, 711.734102)
  line L278 (-73.445218, 711.734102) -> (-73.770204, 711.984063)
  line L279 (-73.770204, 711.984063) -> (-74.020258, 712.309055)
  line L280 (-74.020258, 712.309055) -> (-74.170394, 712.708984)
  line L281 (-74.170394, 712.708984) -> (-74.245268, 713.108391)
  line L282 (-105.245245, 713.108394) -> (-105.170214, 713.534161)
  line L283 (-105.170214, 713.534161) -> (-105.020247, 713.909169)
  line L284 (-105.020247, 713.909169) -> (-104.77027, 714.234177)
  line L285 (-104.77027, 714.234177) -> (-104.445291, 714.484219)
  line L286 (-104.445291, 714.484219) -> (-104.045334, 714.659273)
  line L287 (-104.045334, 714.659273) -> (-103.645324, 714.70929)
  line L288 (-103.645324, 714.70929) -> (-103.245335, 714.65927)
  line L289 (-103.245335, 714.65927) -> (-102.845343, 714.484247)
  line L290 (-102.845343, 714.484247) -> (-102.520335, 714.23427)
  line L291 (-102.520335, 714.23427) -> (-102.270303, 713.909305)
  line L292 (-102.270303, 713.909305) -> (-102.120296, 713.534313)
  line L293 (-102.120296, 713.534313) -> (-102.070277, 713.109272)
  line L294 (-102.070277, 713.109272) -> (-102.120296, 712.709294)
  line L295 (-102.120296, 712.709294) -> (-102.270268, 712.309311)
  line L296 (-102.270268, 712.309311) -> (-102.520266, 711.984276)
  line L297 (-102.520266, 711.984276) -> (-102.84521, 711.73426)
  line L298 (-102.84521, 711.73426) -> (-103.245165, 711.584114)
  line L299 (-103.245165, 711.584114) -> (-103.645165, 711.534098)
  line L300 (-103.645165, 711.534098) -> (-104.045186, 711.584122)
  line L301 (-104.045186, 711.584122) -> (-104.445183, 711.734099)
  line L302 (-104.445183, 711.734099) -> (-104.770183, 711.984071)
  line L303 (-104.770183, 711.984071) -> (-105.020236, 712.309063)
  line L304 (-105.020236, 712.309063) -> (-105.17037, 712.708985)
  line L305 (-105.17037, 712.708985) -> (-105.245245, 713.108394)
  line L306 (-29.317325, 745.634246) -> (-29.323282, 718.434313)
  line L307 (-146.967311, 745.66001) -> (-29.317325, 745.634246)
  line L308 (-146.973268, 718.460078) -> (-146.967311, 745.66001)
  line L309 (-103.657753, 675.125587) -> (-146.973268, 718.460078)
  line L310 (-72.657773, 675.118798) -> (-103.657753, 675.125587)
  line L311 (-29.323282, 718.434313) -> (-72.657773, 675.118798)
  line L312 (-83.995304, 713.059318) -> (-88.145309, 713.609327)
  circle A0 centre (-88.145301, 697.609309) radius 16.000019
  point P0 (0, 0)
  constraints: 1 centre point
sketch "Sketch2 outline for Extrusion2" plane through (0, 0, 0) normal (0, -1, 0) x (1, 0, 0)
  circle A0 centre (-88.145301, 697.609309) radius 16.000019
extrude "Extrusion2" cut sketch "Sketch2 outline for Extrusion2" against normal blind 6
sketch "Sketch3" plane through (0, 0, 0) normal (0, -1, 0) x (1, 0, 0)
  line L0 (-122.920216, 715.584329) -> (-121.370225, 715.809294)
  line L1 (-121.370225, 715.809294) -> (-121.370394, 703.809278)
  circle A0 centre (-121.370309, 709.809286) radius 6
  line L2 (-56.470304, 715.584314) -> (-54.920313, 715.809279)
  line L3 (-53.370281, 704.009266) -> (-54.920295, 703.809281)
  line L4 (-54.920313, 715.809279) -> (-54.920295, 703.809281)
  circle A1 centre (-54.920304, 709.80928) radius 6
  line L5 (-112.845114, 706.634306) -> (-112.445132, 706.709288)
  line L6 (-112.045299, 703.534186) -> (-112.445314, 703.50911)
  line L7 (-112.445132, 706.709288) -> (-112.445314, 703.50911)
  line L8 (-104.045334, 714.659273) -> (-103.645324, 714.70929)
  line L9 (-103.245165, 711.584114) -> (-103.645165, 711.534098)
  line L10 (-103.645324, 714.70929) -> (-103.645165, 711.534098)
  line L11 (-73.045332, 714.659284) -> (-72.645364, 714.709296)
  line L12 (-72.245184, 711.58411) -> (-72.645205, 711.534091)
  line L13 (-72.645364, 714.709296) -> (-72.645205, 711.534091)
  line L14 (-63.845371, 706.709172) -> (-63.445342, 706.63421)
  line L15 (-63.845371, 706.709172) -> (-63.845371, 703.50911)
  line L16 (-104.0429, 683.6591) -> (-103.642836, 683.709124)
  line L17 (-103.242551, 680.583608) -> (-103.642546, 680.533593)
  line L18 (-103.642836, 683.709124) -> (-103.642546, 680.533593)
  line L19 (-72.245919, 680.584234) -> (-72.645863, 680.534224)
  line L20 (-72.645863, 683.711956) -> (-72.645863, 680.534224)
  circle A2 centre (-112.445223, 705.109199) radius 1.6
  circle A3 centre (-103.645245, 713.121694) radius 1.6
  circle A4 centre (-72.645284, 713.121694) radius 1.6
  circle A5 centre (-63.845371, 705.109141) radius 1.6
  circle A6 centre (-72.645863, 682.12309) radius 1.6
  circle A7 centre (-103.642691, 682.121358) radius 1.6
  line L21 (-137.620314, 735.859289) -> (-136.970314, 735.959304)
  line L22 (-136.970367, 730.934291) -> (-136.320343, 731.009311)
  line L23 (-136.970314, 735.959304) -> (-136.970367, 730.934291)
  line L24 (-74.245863, 735.959304) -> (-74.245863, 730.934291)
  line L25 (-39.320302, 735.959314) -> (-38.670302, 735.859299)
  line L26 (-38.670292, 731.009299) -> (-39.320296, 730.934282)
  line L27 (-39.320302, 735.959314) -> (-39.320296, 730.934282)
  circle A8 centre (-136.97034, 733.446797) radius 2.6
  circle A9 centre (-74.245863, 733.446797) radius 2.6
  circle A10 centre (-39.320302, 733.446798) radius 2.6
  line L28 (-146.967311, 745.66001) -> (-29.317325, 745.634246)
  line L29 (-88.142318, 745.647128) -> (-88.142318, 725.299728)
  circle A11 centre (-102.038773, 733.446797) radius 2.6
  point P0 (0, 0)
  dimension "d4" = 12
  dimension "d5" = 12
  dimension "d6" = 3.2
  dimension "d7" = 3.2
  dimension "d8" = 3.2
  dimension "d9" = 3.2
  dimension "d10" = 3.2
  dimension "d11" = 3.2
  dimension "d12" = 5.2
  dimension "d13" = 5.2
  dimension "d14" = 5.2
  constraints: 24 end point, 12 centre point, 12 midpoint, 4 vertical, 1 symmetric about line, 1 other
  measures "d4" diameter of A0
  measures "d5" diameter of A1
  measures "d6" diameter of A2
  measures "d7" diameter of A3
  measures "d8" diameter of A4
  measures "d9" diameter of A5
  measures "d10" diameter of A6
  measures "d11" diameter of A7
  measures "d12" diameter of A8
  measures "d13" diameter of A9
  measures "d14" diameter of A10
sketch "Sketch4" plane through (0, 0, 0) normal (0, -1, 0) x (1, 0, 0)
  point P0 (0, 0)
extrude "Extrusion3" cut sketch "Sketch3" against normal blind 6
body "Solid1"
